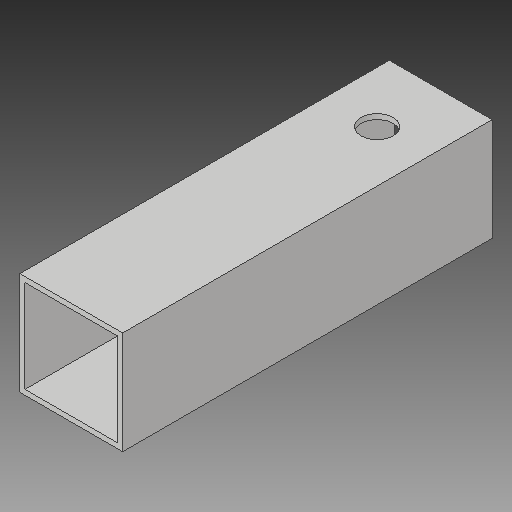
# Autodesk Inventor part: ステア棒
Saved by Autodesk Inventor 2018 (Build 220112000, 112)
## iProperties
Created: 2017-09-20
Part Number: ステア棒
Material: 一般
Document SubType Name: Modeling
Designer: mura5
Density: 1 g/cm^3
Appearance: 既定
Mass: 22.1231 g
Surface Area: 281.435 cm^2
Volume: 22.1231 cm^3
Author: mura5
Autodesk Inventor part; units mm, degrees
ref_plane "YZ Plane" through (0, 0, 0) normal (1, 0, 0) x (0, 1, 0)
ref_plane "XZ Plane" through (0, 0, 0) normal (0, 1, 0) x (-1, 0, 0)
sketch "スケッチ1" plane through (0, 0, 0) normal (0, 1, 0) x (-1, 0, 0)
  line L0 (-901.8, 0) -> (67, 0)
  line L1 (-417.4, -1177.3333) -> (67, 0)
  line L2 (50, -15) -> (50, 15)
  line L3 (24, 15) -> (24, -15)
  line L4 (24, -15) -> (84, -15)
  line L5 (84, 15) -> (84, -15)
  line L6 (-514.28, 15) -> (163.88, 15)
  line L7 (34, 15) -> (34, -80.2064)
  point P0 (0, 0)
  dimension "d0" = 16
  constraints: 16 end point, 2 point on line, 1 horizontal, 1 vertical, 2 other
  measures "d0" distance from line of L2 L7.start
ref_plane "作業平面1" through (514.28, 0, 15) normal (0, 0, 1) x (-1, 0, 0)
sketch "スケッチ2" plane through (514.28, 0, 15) normal (0, 0, 1) x (-1, 0, 0)
  line L0 (0, 0) -> (678.16, 0) projected
  line L1 (532.28, -16) -> (564.28, -16)
  line L2 (564.28, -16) -> (564.28, 16)
  line L3 (564.28, 16) -> (532.28, 16)
  line L4 (532.28, 16) -> (532.28, -16)
  line L5 (532.28, -16) -> (564.28, 16) construction
  line L6 (564.28, -16) -> (532.28, 16) construction
  line L7 (562.68, -14.4) -> (533.88, -14.4)
  line L8 (533.88, -14.4) -> (533.88, 14.4)
  line L9 (533.88, 14.4) -> (562.68, 14.4)
  line L10 (562.68, 14.4) -> (562.68, -14.4)
  point P0 (514.28, 0)
  point P1 (564.28, 0)
  point P2 (564.28, 0)
  point P3 (564.28, 0)
  point P4 (548.28, 0)
  point P5 (548.28, 0)
  point P6 (548.28, 0)
  dimension "d2" = 32
  dimension "d3" = 1.6
  constraints: 20 end point, 4 parallel, 2 midpoint, 2 perpendicular, 1 horizontal, 4 other
  measures "d2" distance of L2.end L1.end
  measures "d3" distance between parallel lines of L1 L7
extrude "押し出し1" add sketch "スケッチ2" against normal blind 115 contours L4 L3 L2 L0 L10 L9 L8 | L0 L8 L7 L10 L2 L1 L4
sketch "スケッチ3" plane through (-50, 16, 15) normal (0, 1, 0) x (1, 0, 0)
  line L0 (467.4, 1192.3333) -> (-17, 15) projected
  line L1 (951.8, 15) -> (-17, 15) projected
  line L2 (16, 0) -> (16, 95.2064) projected
  point P0 (50, 15)
  point P1 (16, 95.2064)
  constraints: 1 coincident
hole "穴1" at (-34, 16, -80.2064) direction (0, -1, 0) diameter 10 end through all
